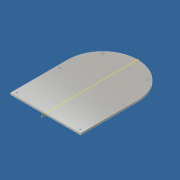
# Autodesk Inventor part: BasePlate_A
Saved by Autodesk Inventor 2016 (Build 200138000, 138)
## iProperties
Created: 2016-02-29
Part Number: BasePlate_A
Material: Aluminium 6061
Document SubType Name: Modeling
Designer: 4ndreas
Density: 2.7 g/cm^3
Appearance: Aluminium - poliert
Mass: 774.553 g
Surface Area: 1198.26 cm^2
Volume: 286.871 cm^3
Author: 4ndreas
Autodesk Inventor part; units mm, degrees
ref_plane "YZ Plane" through (0, 0, 0) normal (1, 0, 0) x (0, 1, 0)
ref_plane "XZ Plane" through (0, 0, 0) normal (0, 1, 0) x (-1, 0, 0)
ref_plane "XY Plane" through (0, 0, 0) normal (0, 0, 1) x (1, 0, 0)
sketch "Skizze1" plane through (0, 0, 0) normal (0, 0, 1) x (1, 0, 0)
  line L0 (-110, -110) -> (110, -110)
  line L1 (110, -110) -> (110, 110)
  line L2 (110, 110) -> (-110, 110)
  line L3 (-110, 110) -> (-110, -110)
  line L4 (-110, -110) -> (110, 110) construction
  line L5 (110, -110) -> (-110, 110) construction
  circle A0 centre (0, 0) radius 95 construction
  circle A1 centre (0, 0) radius 105 construction
  line L6 (-90, 90) -> (-110, 90) construction
  line L7 (-110, 90) -> (-110, 110) construction
  line L8 (-110, 110) -> (-90, 110) construction
  line L9 (-90, 110) -> (-90, 90) construction
  line L10 (-90, 90) -> (-110, 110) construction
  line L11 (-110, 90) -> (-90, 110) construction
  line L12 (110, -110) -> (-110, -110)
  line L13 (-110, -110) -> (-110, -180)
  line L14 (-110, -180) -> (110, -180)
  line L15 (110, -180) -> (110, -110)
  line L16 (90, 90) -> (110, 90) construction
  line L17 (110, 90) -> (110, 110) construction
  line L18 (110, 110) -> (90, 110) construction
  line L19 (90, 110) -> (90, 90) construction
  line L20 (90, 90) -> (110, 110) construction
  line L21 (110, 90) -> (90, 110) construction
  line L22 (90, -160) -> (110, -160) construction
  line L23 (110, -160) -> (110, -180) construction
  line L24 (110, -180) -> (90, -180) construction
  line L25 (90, -180) -> (90, -160) construction
  line L26 (90, -160) -> (110, -180) construction
  line L27 (110, -160) -> (90, -180) construction
  line L28 (-90, -160) -> (-110, -160) construction
  line L29 (-110, -160) -> (-110, -180) construction
  line L30 (-110, -180) -> (-90, -180) construction
  line L31 (-90, -180) -> (-90, -160) construction
  line L32 (-90, -160) -> (-110, -180) construction
  line L33 (-110, -160) -> (-90, -180) construction
  line L34 (-90, -90) -> (-110, -90) construction
  line L35 (-110, -90) -> (-110, -110) construction
  line L36 (-110, -110) -> (-90, -110) construction
  line L37 (-90, -110) -> (-90, -90) construction
  line L38 (-90, -90) -> (-110, -110) construction
  line L39 (-110, -90) -> (-90, -110) construction
  line L40 (90, -90) -> (110, -90) construction
  line L41 (110, -90) -> (110, -110) construction
  line L42 (110, -110) -> (90, -110) construction
  line L43 (90, -110) -> (90, -90) construction
  line L44 (90, -90) -> (110, -110) construction
  line L45 (110, -90) -> (90, -110) construction
  circle A2 centre (0, 0) radius 87.5
  line L46 (110, 45.5635) -> (45.5635, 110) construction
  line L47 (-45.5635, 110) -> (-110, 45.5635) construction
  line L48 (45.5635, 110) -> (-45.5635, 110)
  line L49 (-45.5635, 110) -> (45.5635, 110) construction
  line L50 (45.5635, 110) -> (110, 45.5635) construction
  line L51 (110, 45.5635) -> (110, -45.5635) construction
  line L52 (110, -45.5635) -> (45.5635, -110) construction
  line L53 (45.5635, -110) -> (-45.5635, -110) construction
  line L54 (-45.5635, -110) -> (-110, -45.5635) construction
  line L55 (-110, -45.5635) -> (-110, 45.5635) construction
  line L56 (-110, 45.5635) -> (-45.5635, 110) construction
  line L57 (110, 0) -> (110, 110)
  line L58 (-110, 0) -> (-110, 110)
  line L59 (110, 0) -> (110, 110)
  line L60 (110, 110) -> (-110, 110)
  line L61 (-110, 110) -> (-110, 0)
  arc A3 (110, 0) -> (0, 110) centre (0, 0) ccw
  arc A4 (0, 110) -> (-110, 0) centre (0, 0) ccw
  circle A5 centre (100, -170) radius 18.5 construction
  circle A6 centre (100, -35) radius 18.5 construction
  circle A7 centre (70.7107, 70.7107) radius 18.5 construction
  circle A8 centre (-70.7107, 70.7107) radius 18.5 construction
  circle A9 centre (-100, -35) radius 18.5 construction
  circle A10 centre (0, 0) radius 100 construction
  line L62 (100, -170) -> (100, 100) construction
  line L63 (-100, -170) -> (-100, 100) construction
  line L64 (110, -20) -> (110, 0) construction
  line L65 (110, 0) -> (90, -70) construction
  line L66 (-110, -20) -> (-110, 0) construction
  point P0 (-100, -100)
  point P1 (100, -100)
  dimension "d0" = 190
  dimension "d1" = 10
  dimension "d2" = 220
  dimension "d3" = 20
  dimension "d4" = 70
  dimension "d14" = 175
  dimension "d15" = 45
  dimension "d16" = 45
  dimension "d21" = 37
  dimension "d25" = 10
  dimension "d26" = 145
  dimension "d27" = 145
  dimension "d28" = 10
  dimension "d29" = 200
  constraints: 134 end point, 25 midpoint, 17 parallel, 16 point on line, 11 centre point, 10 coincident, 10 equal length, 9 perpendicular, 8 horizontal, 6 point on circle, 4 collinear, 1 equal radius, 17 other
  measures "d0" diameter of A0
  measures "d1" radial gap between concentric circles of A0 A1
  measures "d2" distance between parallel lines of L0 L2
  measures "d3" distance between parallel lines of L2 L6
  measures "d4" distance between parallel lines of L14 L12
  measures "d14" diameter of A2
  measures "d15" angle of L46 L2
  measures "d16" angle of L47 L2
  measures "d21" diameter of A5
  measures "d25" distance from line of A9.centre L55
  measures "d26" distance from line of L14 A9.centre
  measures "d27" distance from line of point (100, -35) L14
  measures "d28" distance from line of point (100, -35) L1
  measures "d29" diameter of A10
extrude "Extrusion1" add sketch "Skizze1" along normal blind 5 contours L3 A4 A3 L1 L0 | L0 L15 L14 L13 | L3 L2 A4 | A3 L2 L1 | A2
hole "Bohrung1" at (100, -170, 0) at (-100, -170, 0) at (-100, 100, 0) at (100, 100, 0) at (-100, -35, 0) at (-70.7107, 70.7107, 0) at (70.7107, 70.7107, 0) at (100, -35, 0) direction (0, 0, 1) diameter 5.3 end through all
sketch "Skizze2" plane through (0, 0, 5) normal (0, 0, 1) x (1, 0, 0)
  circle A0 centre (-100, 100) radius 2.65 projected
  circle A1 centre (100, -170) radius 2.65 projected
  circle A2 centre (-100, -170) radius 2.65 projected
  circle A3 centre (100, 100) radius 2.65 projected
  line L0 (-110, 110) -> (-110, -180) projected
  line L1 (-110, -180) -> (110, -180) projected
  line L2 (110, -180) -> (110, 110) projected
  line L3 (110, 110) -> (-110, 110) projected
  arc A4 (110, 0) -> (-110, 0) centre (0, 0) ccw
  line L4 (110, -180) -> (110, 110) projected
  line L5 (-110, 110) -> (-110, -180) projected
  line L6 (110, 110) -> (-110, 110) projected
  dimension "d22" = 50
  dimension "d23" = 35
  constraints: 2 point on circle, 2 point on line, 1 centre point, 1 coincident, 1 tangent
extrude "Extrusion3" cut sketch "Skizze2" against normal through all contours L3 A4 L0 | L3 L2 A4
ref_plane "Arbeitsebene1" through (0, -180, 0) normal (-1, 0, 0) x (0, 0, 1)
equation "\"d16\" = d15"
equation "\"d27\" = d26"
equation "\"d28\" = d25"
